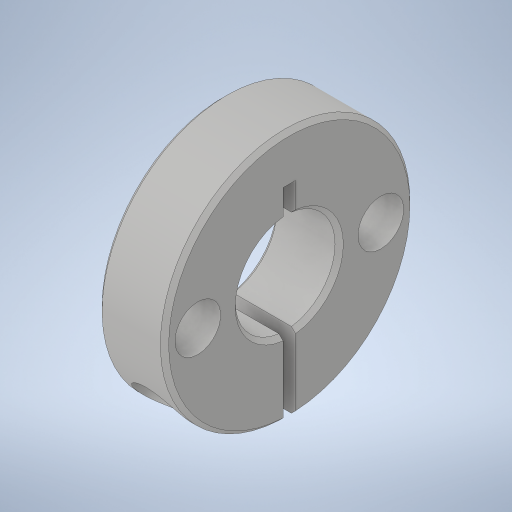
# Autodesk Inventor part: SSCSM12-8b
Saved by Autodesk Inventor 2023.2 (Build 272271030, 271C)
## iProperties
Created: 2023-04-27
Part Number: SSCSM12-8b
Material: Generic
Catalog Web Link: www.cadenas.de
Description: SCSM, PSCSM, SSCSM, SCSMA, SCSMAW-b-Set Collars - Slit 2 Hole/2 Tap - Standard Type - 2 Hole Type
Vendor: MISUMI
Document SubType Name: Modeling
Designer: psAdmin
Manufacturer: MISUMI
Mass: 3.93022 g
Surface Area: 26.8096 cm^2
Volume: 3.93022 cm^3
Density: 1 g/cm^3
Appearance: PSOLRGB-175-175-175
Category: PARTsolutions
Company: MISUMI
PSOL_IDENT_0: {$CADENAS_DATA/23d-libs/misumi/metric/03_set_collars/scsm_b.prj},200 {VTYP=3D},{NB=SSCSM12-8b},{LINA=
PSOL_IDENT_1: SSCSM12-8b},{NN=SCSM, PSCSM, SSCSM, SCSMA, SCSMAW-b},{DATE=30.11.2021 05:42:00},{GEOMDATE=15.09.2021
PSOL_IDENT_2: 05:24:18},{VERSION=},{LINEID=70},{WBVAR=MAT,ST,BS},{WBNUMERIC=BS}  {NB=SSCSM12-8b},{LINA=SSCSM12-8b
PSOL_IDENT_3: },{KT=DUMMY},{PN=SSCSM12-8},{TYPE=SSCSM},{MAT=304},{ST=-},{ST0='-','-'},{AC=Hexagon Socket Head Set
PSOL_IDENT_4: Screw 1 Pc. (304 Stainless Steel) },{D=12},{BS=8},{B1=8,10,12,15},{D1=30},{M=M3},{THMD=3},{THDMIN=2.
PSOL_IDENT_5: 459},{DD=3.4},{R=3.00},{W=1.5},{X=10.0},{Y=5.0},{Z=9~10},{S=5.5},{P=22},{C=0.5},{L=12},{M1=-},{ZZ=9.
PSOL_IDENT_6: 5},{MATA='1045','S45C Equivalent','304','SUS304 Equivalent','2017','2017 Aluminum Alloy'}
NB: SSCSM12-8b
NN: SCSM, PSCSM, SSCSM, SCSMA, SCSMAW-b
NT: Set Collars - Slit 2 Hole/2 Tap - Standard Type - 2 Hole Type
NBSYN: $PN.b
LINA: SSCSM12-8b
CATALOG: Misumi
PN: SSCSM12-8
MAT: SUS304 Equivalent
ST: -
AC: Hexagon Socket Head Set Screw 1 Pc. (304 Stainless Steel)
D: 12
BS: 8
D1: 30
M: M3
DD: 3.4
R: 3
W: 1.5
X: 10
Y: 5
Z: 9~10
S: 5.5
P: 22
SUPPLIER: MISUMI
ARTICLENO: SSCSM12-8b
BOMINFO: SSCSM12-8b
CREATOR: CADENAS GmbH
Title: SSCSM12-8b
Author: Cadenas PARTsolutions
Comments: Set Collars - Slit 2 Hole/2 Tap - Standard Type - 2 Hole Type
Autodesk Inventor part; units mm, degrees
sketch "Sketch_1" plane through (0, 0, 0) normal (0, 0, 1) x (1, 0, 0)
  line L0 (4, 0) -> (-4, 0)
  line L1 (-4, 14.5) -> (-4, 6.5)
  line L2 (-4, 6.5) -> (-3.5, 6)
  line L3 (-3.5, 6) -> (3.5, 6)
  line L4 (3.5, 6) -> (4, 6.5)
  line L5 (4, 6.5) -> (4, 14.5)
  line L6 (4, 14.5) -> (3.5, 15)
  line L7 (3.5, 15) -> (-3.5, 15)
  line L8 (-3.5, 15) -> (-4, 14.5)
  constraints: 18 end point
revolve "Revolution1" add sketch "Sketch_1" angle 360 about axis through (4, 0, 0) along (1, 0, 0)
sketch "Sketch_2" plane through (0, 0, 0) normal (1, 0, 0) x (0, 1, 0)
  line L0 (-15, 0.75) -> (-15, -0.75)
  line L1 (-15, -0.75) -> (9.5, -0.75)
  line L2 (9.5, -0.75) -> (9.5, 0.75)
  line L3 (9.5, 0.75) -> (-15, 0.75)
  constraints: 8 end point
extrude "Extrusion1" cut sketch "Sketch_2" along normal mid plane 8
sketch "Sketch_3" plane through (0, 0, 0) normal (1, 0, 0) x (0, 1, 0)
  line L0 (-10, 15) -> (-10, 0)
  line L1 (-10, 0) -> (-11.7, 0)
  line L2 (-11.7, 0) -> (-11.7, 5)
  line L3 (-11.7, 5) -> (-13, 5)
  line L4 (-13, 5) -> (-13, 15)
  line L5 (-13, 15) -> (-10, 15)
  line L6 (-10, 15) -> (-10, 0)
  constraints: 14 end point
revolve "Revolution2" cut sketch "Sketch_3" angle 360 about axis through (0, -10, 15) along (0, 0, 1)
sketch "Sketch_4" plane through (0, 0, 0) normal (1, 0, 0) x (0, 1, 0)
  line L0 (-10, -15.75) -> (-10, -0.75)
  line L1 (-10, -0.75) -> (-8.5, -0.75)
  line L2 (-8.5, -0.75) -> (-8.7705, -1.0205)
  line L3 (-8.7705, -1.0205) -> (-8.7705, -15.75)
  line L4 (-8.7705, -15.75) -> (-10, -15.75)
  line L5 (-10, -15.75) -> (-10, -0.75)
  constraints: 12 end point
revolve "Revolution3" cut sketch "Sketch_4" angle 360 about axis through (0, -10, -15.75) along (0, 0, -1)
thread "Thread1" size "M3x0.5" class "6H" standard "ISO Metric profile" length 11.3387
sketch "Sketch_7" plane through (0, 0, 0) normal (1, 0, 0) x (0, 1, 0)
  circle A0 centre (0, -11) radius 2.75
  constraints: 1 centre point
extrude "Extrusion2" cut sketch "Sketch_7" along normal mid plane 16
sketch "Sketch_8" plane through (0, 0, 0) normal (1, 0, 0) x (0, 1, 0)
  circle A0 centre (0, 11) radius 2.75
  constraints: 1 centre point
extrude "Extrusion3" cut sketch "Sketch_8" along normal mid plane 16
ref_plane "body_screw_XY" through (0, -10, 5) normal (0, 0, 1) x (1, 0, 0)
ref_plane "body_screw_YZ" through (0, -10, 5) normal (1, 0, 0) x (0, 1, 0)
ref_plane "body_screw_ZX" through (0, -10, 5) normal (0, 1, 0) x (0, 0, 1)
body "Solid1"
